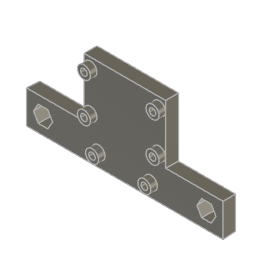
cam and tof holder (Autodesk Fusion 360 design; units mm, degrees)
Autodesk Fusion 360 part; units mm, degrees
sketch "Sketch1" plane through (0, 0, 0) normal (0, 1, 0) x (1, 0, 0)
  line L0 (12.5, 9) -> (-12.5, 9)
  line L1 (-12.5, 9) -> (-12.5, -9)
  line L2 (-12.5, -9) -> (12.5, -9)
  line L3 (12.5, -9) -> (12.5, 9)
  line L4 (12.5, 9) -> (-12.5, -9) construction
  line L5 (-12.5, 9) -> (12.5, -9) construction
  line L6 (10.5, 6) -> (-10.5, 6) construction
  line L7 (-10.5, 6) -> (-10.5, -6) construction
  line L8 (-10.5, -6) -> (10.5, -6) construction
  line L9 (10.5, -6) -> (10.5, 6) construction
  line L10 (10.5, 6) -> (-10.5, -6) construction
  line L11 (-10.5, 6) -> (10.5, -6) construction
  circle A0 centre (-10.5, -6) radius 1
  circle A1 centre (-10.5, -6) radius 2
  circle A2 centre (10.5, -6) radius 1
  circle A3 centre (10.5, -6) radius 2
  circle A4 centre (-10.5, 6) radius 1
  circle A5 centre (-10.5, 6) radius 2
  circle A6 centre (10.5, 6) radius 1
  circle A7 centre (10.5, 6) radius 2
  dimension "d1" = 25
  dimension "d2" = 18
  dimension "d3" = 21
  dimension "d4" = 12
  dimension "d5" = 2
  dimension "d6" = 4
  dimension "d7" = 2
  dimension "d8" = 4
  dimension "d9" = 2
  dimension "d10" = 4
  dimension "d11" = 2
  dimension "d12" = 4
  constraint horizontal L0
  constraint perpendicular L0 L1
  constraint parallel L0 L2
  constraint parallel L1 L3
  constraint coincident L4 origin
  constraint coincident L5 origin
  constraint horizontal L6
  constraint perpendicular L6 L7
  constraint parallel L6 L8
  constraint parallel L7 L9
  constraint coincident L10 origin
  constraint coincident L11 origin
  constraint coincident L7.end L8.start
  constraint concentric A0 A1
  constraint coincident L8.end L9.start
  constraint concentric A2 A3
  constraint coincident L6.end L7.start
  constraint concentric A4 A5
  constraint coincident L6.start L9.end
  constraint concentric A6 A7
  measures "d1" distance of L1.end L2.end
  measures "d2" distance of L0.end L1.end
  measures "d3" distance of L7.end L8.end
  measures "d4" distance of L6.end L7.end
  measures "d5" diameter of A0
  measures "d6" diameter of A1
  measures "d7" diameter of A2
  measures "d8" diameter of A3
  measures "d9" diameter of A4
  measures "d10" diameter of A5
  measures "d11" diameter of A6
  measures "d12" diameter of A7
extrude "Extrude1" add sketch "Sketch1" along normal blind 2 contours A5 | A1 | A3 | A7 | L0 L1 L2 L3 | A0 | A2 | A4 | A6
extrude "Extrude2" add sketch "Sketch1" against normal blind 2 contours A5 | A1 | A3 | A7
move_face "OffsetFaces1" offset 10 1 faces at (4.1667, 0.6667, -9)
sketch "Sketch2" plane through (0, 0, 0) normal (0, -1, 0) x (1, 0, 0)
  circle A0 centre (-10.5, -6) radius 2
  line L0 (-12.5, -19) -> (12.5, -19)
  circle A1 centre (10.5, -6) radius 2
  line L1 (-12.5, 6) -> (-12.5, -6)
  line L2 (-12.5, -6) -> (-12.5, -19)
  line L3 (12.5, -19) -> (12.5, -6)
  line L4 (12.5, -6) -> (12.5, 6)
  line L5 (12.5, -19) -> (-12.5, -19)
  line L6 (-12.5, -19) -> (-12.5, -11)
  line L7 (-12.5, -11) -> (12.5, -11)
  line L8 (12.5, -11) -> (12.5, -19)
  line L9 (-12.5, -19) -> (12.5, -11) construction
  line L10 (-8, -15) -> (8, -15) construction
  circle A2 centre (-8, -15) radius 1
  circle A3 centre (-8, -15) radius 2
  circle A4 centre (8, -15) radius 1
  circle A5 centre (8, -15) radius 2
  point P0 (0, -15)
  dimension "d38" = 8
  dimension "d39" = 16
  dimension "d40" = 2
  dimension "d41" = 4
  dimension "d42" = 2
  dimension "d43" = 4
  constraint horizontal L5
  constraint vertical L6
  constraint horizontal L7
  constraint vertical L8
  constraint coincident L2 L6.end
  constraint coincident L0.end L3.start
  constraint midpoint L10 P0
  constraint coincident L9 P0
  constraint parallel L7 L10
  constraint coincident L10.start A2.centre
  constraint concentric A2 A3
  constraint midpoint L9 P0
  constraint coincident L10.end A4.centre
  constraint concentric A4 A5
  measures "d38" distance of L0.end L7.end
  measures "d39" distance of L10.start L10.end
  measures "d40" diameter of A2
  measures "d41" diameter of A3
  measures "d42" diameter of A4
  measures "d43" diameter of A5
extrude "Extrude3" add sketch "Sketch2" along normal blind 2 contours A3 | A5
sketch "Sketch3" plane through (0, 2, 0) normal (0, 1, 0) x (-1, 0, 0)
  line L0 (-12.5, 9) -> (-12.5, -19)
  line L1 (-12.5, -19) -> (12.5, -19)
  line L2 (12.5, -19) -> (12.5, 9)
  line L3 (12.5, 9) -> (-12.5, 9)
  line L4 (-30, -9) -> (30, -9)
  line L5 (30, -9) -> (30, -19)
  line L6 (30, -19) -> (-30, -19)
  line L7 (-30, -19) -> (-30, -9)
  line L8 (-30, -9) -> (30, -19) construction
  line L9 (-25, -14) -> (25, -14) construction
  line L10 (-23.4989, -16.6) -> (-21.9978, -14)
  line L11 (-21.9978, -14) -> (-23.4989, -11.4)
  line L12 (-23.4989, -11.4) -> (-26.5011, -11.4)
  line L13 (-26.5011, -11.4) -> (-28.0022, -14)
  line L14 (-28.0022, -14) -> (-26.5011, -16.6)
  line L15 (-26.5011, -16.6) -> (-23.4989, -16.6)
  line L16 (28.0022, -14) -> (26.5011, -11.4)
  line L17 (26.5011, -11.4) -> (23.4989, -11.4)
  line L18 (23.4989, -11.4) -> (21.9978, -14)
  line L19 (21.9978, -14) -> (23.4989, -16.6)
  line L20 (23.4989, -16.6) -> (26.5011, -16.6)
  line L21 (26.5011, -16.6) -> (28.0022, -14)
  point P0 (0, -14)
  point P1 (-25, -14)
  point P2 (25, -14)
  dimension "d27" = 60
  dimension "d28" = 10
  dimension "d29" = 50
  dimension "d30" = 2.6
  dimension "d31" = 2.6
  constraint horizontal L4
  constraint vertical L5
  constraint horizontal L6
  constraint vertical L7
  constraint midpoint L1 L6
  constraint midpoint L9 P0
  constraint coincident L8 P0
  constraint perpendicular L2 L9
  constraint midpoint L8 P0
  constraint coincident P1 L9.start
  constraint horizontal L15
  constraint coincident P2 L9.end
  constraint horizontal L20
  measures "d27" distance of L4.start L4.end
  measures "d28" distance of L4.start L6.end
  measures "d29" distance of P1 P2
  measures "d30" distance of P1 L15
  measures "d31" distance of P2 L21
extrude "Extrude4" add sketch "Sketch3" against normal blind 2 draft 2 contours L0 L1 L2 L4 L6 | L0 L4 L6 L7 | L2 L4 L5 L6
move_face "OffsetFaces2" offset 2 1 faces at (-4.1667, 2, 3)
fillet "Fillet1" [suppressed]
named bodies: "front plate"
